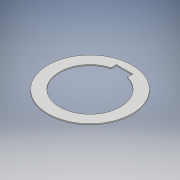
# Autodesk Inventor part: 軸心墊片
Saved by Autodesk Inventor 2018 (Build 220112000, 112)
## iProperties
Created: 2025-05-19
Part Number: 軸心墊片
Material: 一般
Document SubType Name: Modeling
Designer: User
Density: 1 g/cm^3
Appearance: 預設
Author: User
Autodesk Inventor part; units mm, degrees
ref_plane "YZ Plane" through (0, 0, 0) normal (1, 0, 0) x (0, 1, 0)
ref_plane "XZ Plane" through (0, 0, 0) normal (0, 1, 0) x (-1, 0, 0)
ref_plane "XY Plane" through (0, 0, 0) normal (0, 0, 1) x (1, 0, 0)
sketch "草圖1" plane through (0, 0, 0) normal (0, 0, 1) x (1, 0, 0)
  circle A0 centre (0, 0) radius 22.5
  circle A1 centre (0, 0) radius 31
  dimension "d0" = 45
  dimension "d1" = 62
  constraints: 2 centre point, 2 coincident
  measures "d0" diameter of A0
  measures "d1" diameter of A1
extrude "擠出1" add sketch "草圖1" along normal blind 0.8
sketch "草圖2" plane through (0, 0, 0.8) normal (0, 0, 1) x (1, 0, 0)
  line L0 (-6.1, 25.6) -> (6.1, 25.6)
  line L1 (6.1, 25.6) -> (6.1, 13.8504)
  line L2 (6.1, 13.8504) -> (-6.1, 13.8504)
  line L3 (-6.1, 13.8504) -> (-6.1, 25.6)
  point P0 (0, 0)
  dimension "d5" = 6.1
  dimension "d6" = 12.2
  dimension "d7" = 25.6
  constraints: 8 end point, 2 parallel, 1 horizontal, 1 perpendicular
  measures "d5" distance from line of point (0, 0) L1
  measures "d6" distance between parallel lines of L1 L3
  measures "d7" distance from line of point (0, 0) L0
extrude "擠出2" cut sketch "草圖2" against normal blind 0.8
